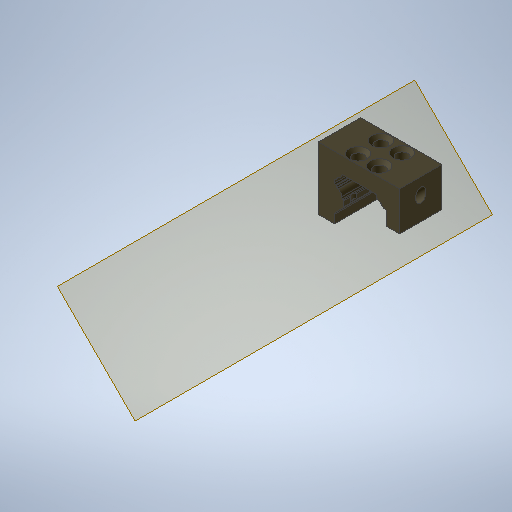
# Autodesk Inventor part: HGR_LIMITSWITCHHOLDER
Saved by Autodesk Inventor 2025.2 (Build 292293000, 293)
## iProperties
Created: 2026-03-18
Part Number: HGR_LIMITSWITCHHOLDER
Material: Generic
Document SubType Name: Modeling
Designer: composite
Density: 1 g/cm^3
Appearance: Default
Author: composite
Autodesk Inventor part; units mm, degrees
ref_plane "YZ Plane" through (0, 0, 0) normal (1, 0, 0) x (0, 1, 0)
ref_plane "XZ Plane" through (0, 0, 0) normal (0, 1, 0) x (-1, 0, 0)
ref_plane "XY Plane" through (0, 0, 0) normal (0, 0, 1) x (1, 0, 0)
derived "HGR15_REPRESENTATIVE.ipt"
sketch "hgr15 REP SKETCH" plane through (-6.8, 0, 100) normal (0, 0, 1) x (1, 0, 0)
  arc A0 (-0.4071, 3.9505) -> (-0.7, 3.2434) centre (0.3, 3.2434) ccw
  line L0 (-0.7, 3.2434) -> (-0.7, 0.7)
  line L1 (-0.7, 0.7) -> (0, 0)
  line L2 (0, 0) -> (13.6, 0)
  line L3 (13.6, 0) -> (14.3, 0.7)
  line L4 (14.3, 0.7) -> (14.3, 3.2434)
  arc A1 (14.3, 3.2434) -> (14.0071, 3.9505) centre (13.3, 3.2434) ccw
  line L5 (14.0071, 3.9505) -> (11.6872, 6.2704)
  arc A2 (11.57, 6.5533) -> (11.6872, 6.2704) centre (11.97, 6.5533) ccw
  line L6 (11.57, 6.5533) -> (11.57, 8.1153)
  arc A3 (11.6872, 8.3982) -> (11.57, 8.1153) centre (11.97, 8.1153) ccw
  line L7 (11.6872, 8.3982) -> (11.8816, 8.5926)
  arc A4 (11.8816, 8.5926) -> (12.0706, 9.0718) centre (11.6914, 8.9445) ccw
  arc A5 (13.2785, 10.4123) -> (12.0706, 9.0718) centre (13.6562, 8.8576) ccw
  arc A6 (13.2785, 10.4123) -> (13.5743, 10.7128) centre (13.1841, 10.801) ccw
  line L8 (13.5743, 10.7128) -> (13.6062, 10.8541)
  arc A7 (13.8606, 11.1421) -> (13.6062, 10.8541) centre (13.9964, 10.7658) ccw
  line L9 (13.8606, 11.1421) -> (14.0357, 11.2052)
  arc A8 (14.0357, 11.2052) -> (14.3, 11.5815) centre (13.9, 11.5815) ccw
  line L10 (14.3, 11.5815) -> (14.3, 12.3375)
  arc A9 (14.3, 12.3375) -> (14.0187, 12.7195) centre (13.9, 12.3375) ccw
  line L11 (14.0187, 12.7195) -> (13.8777, 12.7633)
  arc A10 (13.6053, 13.0612) -> (13.8777, 12.7633) centre (13.9964, 13.1453) ccw
  line L12 (13.6053, 13.0612) -> (13.575, 13.2021)
  arc A11 (13.575, 13.2021) -> (13.2784, 13.5067) centre (13.184, 13.118) ccw
  arc A12 (12.074, 14.8234) -> (13.2784, 13.5067) centre (13.6562, 15.0614) ccw
  arc A13 (12.074, 14.8234) -> (11.8861, 14.9629) centre (11.7521, 14.586) ccw
  line L13 (11.8861, 14.9629) -> (11.849, 15)
  line L14 (11.849, 15) -> (1.751, 15)
  line L15 (1.751, 15) -> (1.7139, 14.9629)
  arc A14 (1.7139, 14.9629) -> (1.526, 14.8234) centre (1.8479, 14.586) ccw
  arc A15 (0.3216, 13.5067) -> (1.526, 14.8234) centre (-0.0562, 15.0614) ccw
  arc A16 (0.3216, 13.5067) -> (0.025, 13.2021) centre (0.416, 13.118) ccw
  line L16 (0.025, 13.2021) -> (-0.0053, 13.0612)
  arc A17 (-0.2777, 12.7633) -> (-0.0053, 13.0612) centre (-0.3964, 13.1453) ccw
  line L17 (-0.2777, 12.7633) -> (-0.4187, 12.7195)
  arc A18 (-0.4187, 12.7195) -> (-0.7, 12.3375) centre (-0.3, 12.3375) ccw
  line L18 (-0.7, 12.3375) -> (-0.7, 11.5815)
  arc A19 (-0.7, 11.5815) -> (-0.4357, 11.2052) centre (-0.3, 11.5815) ccw
  line L19 (-0.4357, 11.2052) -> (-0.2606, 11.1421)
  arc A20 (-0.0062, 10.8541) -> (-0.2606, 11.1421) centre (-0.3964, 10.7658) ccw
  line L20 (-0.0062, 10.8541) -> (0.0257, 10.7128)
  arc A21 (0.0257, 10.7128) -> (0.3215, 10.4123) centre (0.4159, 10.801) ccw
  arc A22 (1.5294, 9.0718) -> (0.3215, 10.4123) centre (-0.0562, 8.8576) ccw
  arc A23 (1.5294, 9.0718) -> (1.7184, 8.5926) centre (1.9086, 8.9445) ccw
  line L21 (1.7184, 8.5926) -> (1.9128, 8.3982)
  arc A24 (2.03, 8.1153) -> (1.9128, 8.3982) centre (1.63, 8.1153) ccw
  line L22 (2.03, 8.1153) -> (2.03, 6.5533)
  arc A25 (1.9128, 6.2704) -> (2.03, 6.5533) centre (1.63, 6.5533) ccw
  line L23 (1.9128, 6.2704) -> (-0.4071, 3.9505)
  point P0 (6.8, 0)
sketch "Sketch2" plane through (0, 0, 0) normal (0, 0, 1) x (1, 0, 0)
  line L0 (-7.5, 3.2434) -> (-7.5, 0.7) projected
  arc A0 (-7.2071, 3.9505) -> (-7.5, 3.2434) centre (-6.5, 3.2434) ccw projected
  line L1 (-5.049, 15) -> (-5.0861, 14.9629) projected
  arc A1 (-5.0861, 14.9629) -> (-5.274, 14.8234) centre (-4.9521, 14.586) ccw projected
  arc A2 (-6.4784, 13.5067) -> (-6.775, 13.2021) centre (-6.384, 13.118) ccw projected
  arc A3 (-6.4784, 13.5067) -> (-5.274, 14.8234) centre (-6.8562, 15.0614) ccw projected
  line L2 (-6.775, 13.2021) -> (-6.8053, 13.0612) projected
  arc A4 (-5.2706, 9.0718) -> (-5.0816, 8.5926) centre (-4.8914, 8.9445) ccw projected
  line L3 (-5.0816, 8.5926) -> (-4.8872, 8.3982) projected
  arc A5 (-4.77, 8.1153) -> (-4.8872, 8.3982) centre (-5.17, 8.1153) ccw projected
  line L4 (-4.77, 8.1153) -> (-4.77, 6.5533) projected
  arc A6 (-4.8872, 6.2704) -> (-4.77, 6.5533) centre (-5.17, 6.5533) ccw projected
  line L5 (-4.8872, 6.2704) -> (-7.2071, 3.9505) projected
  arc A7 (-7.0777, 12.7633) -> (-6.8053, 13.0612) centre (-7.1964, 13.1453) ccw projected
  line L6 (-7.0777, 12.7633) -> (-7.2187, 12.7195) projected
  line L7 (-6.8062, 10.8541) -> (-6.7743, 10.7128) projected
  arc A8 (-6.7743, 10.7128) -> (-6.4785, 10.4123) centre (-6.3841, 10.801) ccw projected
  arc A9 (-7.2187, 12.7195) -> (-7.5, 12.3375) centre (-7.1, 12.3375) ccw projected
  line L8 (-7.2357, 11.2052) -> (-7.0606, 11.1421) projected
  line L9 (-7.5, 12.3375) -> (-7.5, 11.5815) projected
  arc A10 (-7.5, 11.5815) -> (-7.2357, 11.2052) centre (-7.1, 11.5815) ccw projected
  arc A11 (-5.2706, 9.0718) -> (-6.4785, 10.4123) centre (-6.8562, 8.8576) ccw projected
  arc A12 (-6.8062, 10.8541) -> (-7.0606, 11.1421) centre (-7.1964, 10.7658) ccw projected
  line L10 (4.77, 6.5533) -> (4.77, 8.1153) construction
  arc A13 (4.77, 6.5533) -> (4.8872, 6.2704) centre (5.17, 6.5533) ccw construction
  arc A14 (4.8872, 8.3982) -> (4.77, 8.1153) centre (5.17, 8.1153) ccw construction
  line L11 (4.8872, 8.3982) -> (5.0816, 8.5926) construction
  arc A15 (5.0816, 8.5926) -> (5.2706, 9.0718) centre (4.8914, 8.9445) ccw construction
  line L12 (7.2187, 12.7195) -> (7.0777, 12.7633) projected
  arc A16 (7.5, 12.3375) -> (7.2187, 12.7195) centre (7.1, 12.3375) ccw projected
  arc A17 (6.8053, 13.0612) -> (7.0777, 12.7633) centre (7.1964, 13.1453) ccw projected
  line L13 (6.8053, 13.0612) -> (6.775, 13.2021) projected
  arc A18 (6.775, 13.2021) -> (6.4784, 13.5067) centre (6.384, 13.118) ccw projected
  arc A19 (5.274, 14.8234) -> (6.4784, 13.5067) centre (6.8562, 15.0614) ccw projected
  arc A20 (5.274, 14.8234) -> (5.0861, 14.9629) centre (4.9521, 14.586) ccw projected
  line L14 (5.0861, 14.9629) -> (5.049, 15) projected
  line L15 (7.5, 11.5815) -> (7.5, 12.3375) construction
  arc A21 (7.2357, 11.2052) -> (7.5, 11.5815) centre (7.1, 11.5815) ccw construction
  line L16 (7.0606, 11.1421) -> (7.2357, 11.2052) construction
  arc A22 (7.0606, 11.1421) -> (6.8062, 10.8541) centre (7.1964, 10.7658) ccw construction
  line L17 (6.7743, 10.7128) -> (6.8062, 10.8541) construction
  arc A23 (6.4785, 10.4123) -> (6.7743, 10.7128) centre (6.3841, 10.801) ccw construction
  arc A24 (6.4785, 10.4123) -> (5.2706, 9.0718) centre (6.8562, 8.8576) ccw construction
  line L18 (5.049, 15) -> (-5.049, 15) projected
  line L19 (-7.5, 0.7) -> (-12.5, 0.7)
  line L20 (-12.5, 0.7) -> (-12.5, 20)
  line L21 (-12.5, 20) -> (12.5, 20)
  line L22 (12.5, 20) -> (12.5, 8)
  line L23 (12.5, 8) -> (8.5, 8)
  line L24 (8.5, 8) -> (8.5, 12.3375)
  line L25 (8.5, 12.3375) -> (7.5, 12.3375)
  point P0 (0, 0)
  dimension "d1" = 5
  dimension "d2" = 5
  dimension "d3" = 4
  dimension "d4" = 12
  dimension "d5" = 1
  constraints: 14 end point, 6 perpendicular, 1 horizontal
  measures "d1" distance of L0.end L19.end
  measures "d2" distance between parallel lines of L21 L18
  measures "d3" distance between parallel lines of L24 L22
  measures "d4" distance between parallel lines of L21 L23
  measures "d5" distance of L24.end L15.end
extrude "Extrusion1" add sketch "Sketch2" along normal blind 13
ref_plane "Work Plane1" through (12.5, 20, 0) normal (0.7071068, 0.7071068, 0) x (0, 0, 1)
sketch "Sketch3" plane through (12.5, 20, 0) normal (0.7071068, 0.7071068, 0) x (0, 0, 1)
  circle A0 centre (6.5, 3.4853) radius 1.5457
  line L0 (0, 8.4853) -> (13, 8.4853) projected
  line L1 (6.5, 8.4853) -> (6.5, 3.4853) construction
  point P0 (0, 5.3033)
  dimension "d9" = 5
  constraints: 2 end point, 1 centre point, 1 midpoint, 1 vertical
  measures "d9" distance from line of L1.end L0
extrude "Extrusion2" cut sketch "Sketch3" against normal blind 13
sketch "Sketch4" plane through (-12.5, 20, 0) normal (0, 1, 0) x (1, 0, 0)
  circle A0 centre (9.25, -10) radius 1.75
  circle A1 centre (15.75, -10) radius 1.75
  circle A2 centre (9.25, -3) radius 1.75
  circle A3 centre (15.75, -3) radius 1.75
  line L0 (25, -13) -> (0, -13) projected
  line L1 (12.5, -13) -> (12.5, 0) construction
  line L2 (7.451, 0) -> (17.549, 0) projected
  line L3 (9.25, -3) -> (12.5, -3) construction
  line L4 (15.75, -3) -> (12.5, -3) construction
  point P0 (12.5, 0)
  dimension "d12" = 3.5
  dimension "d13" = 3.5
  dimension "d14" = 3.5
  dimension "d15" = 3.5
  dimension "d16" = 6.5
  dimension "d19" = 3
  dimension "d20" = 3
  constraints: 6 end point, 4 centre point, 2 horizontal alignment, 2 midpoint, 2 vertical alignment, 1 collinear, 1 horizontal, 1 perpendicular, 1 point on line, 1 vertical
  measures "d12" diameter of A0
  measures "d13" diameter of A2
  measures "d14" diameter of A3
  measures "d15" diameter of A1
  measures "d16" distance of L4.start L3.start
  measures "d19" distance from line of L3.start L2
  measures "d20" distance from line of L0 A0.centre
extrude "Extrusion3" cut sketch "Sketch4" against normal blind 13
chamfer "Chamfer1" distance 1 angle 45 4 edges at (-5, 20, 10) (-5, 20, 3) (1.5, 20, 3) (1.5, 20, 10)
equation "\"d13\" = d12"
equation "\"d14\" = d12"
equation "\"d15\" = d12"
equation "\"d20\" = d19"
body "Solid1"
